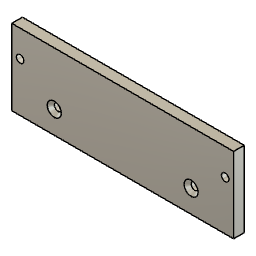
tip top audio zrail bracket (Autodesk Fusion 360 design; units mm, degrees)
Autodesk Fusion 360 part; units mm, degrees
note: some values were not read from the file. Set by a fixed rule: the direction of a hole.
sketch "Sketch2" plane through (0, 0, 0) normal (0, 0, 1) x (1, 0, 0)
  line L0 (-66.2534, 12.7) -> (66.2534, 12.7)
  line L1 (66.2534, 12.7) -> (66.2534, -12.7)
  line L2 (66.2534, -12.7) -> (-66.2534, -12.7)
  line L3 (-66.2534, -12.7) -> (-66.2534, 12.7)
  line L4 (-66.2534, 0) -> (66.2534, 0) construction
  line L5 (0, 12.7) -> (0, -12.7) construction
  line L6 (-66.2534, -12.7) -> (66.2534, -12.7)
  line L7 (66.2534, -12.7) -> (66.2534, -32.512)
  line L8 (66.2534, -32.512) -> (-66.2534, -32.512)
  line L9 (-66.2534, -32.512) -> (-66.2534, -12.7)
  point P0 (-61.2521, 0)
  point P1 (61.2521, 0)
  point P2 (-40.8534, -19.05)
  point P3 (-61.2521, -3.2004)
  point P4 (61.2521, -3.2004)
  point P5 (40.8534, -19.05)
  dimension "d2" = 25.4
  dimension "d3" = 122.5042
  dimension "d4" = 132.5067
  dimension "d18" = 3.2004
  dimension "d19" = 25.4
  dimension "d22" = 19.05
  dimension "d23" = 19.812
  constraint horizontal L0
  constraint vertical L1
  constraint horizontal L2
  constraint vertical L3
  constraint horizontal P0 P1
  constraint midpoint L3 L4.start
  constraint midpoint L1 L4.end
  constraint coincident P1 L4
  constraint midpoint L0 L5.start
  constraint midpoint L2 L5.end
  constraint symmetric P0 P1 L5
  constraint midpoint L4 origin
  constraint horizontal P3 P4
  constraint vertical P1 P4
  constraint vertical P0 P3
  constraint horizontal L6
  constraint vertical L7
  constraint horizontal L8
  constraint vertical L9
  constraint coincident L2.end L3.start
  constraint collinear L1 L7
  constraint symmetric L5 P2 P5
  measures "d2" distance of L0.start L2.end
  measures "d3" distance of P0 P1
  measures "d4" distance of L0.start L0.end
  measures "d18" distance of P0 P3
  measures "d19" distance of L3 P2
  measures "d22" distance of L4 P2
  measures "d23" distance of L6 L8
extrude "Extrude1" add sketch "Sketch2" along normal blind 6.35
hole "Hole1" at (-61.2521, -3.2004, 0) at (61.2521, -3.2004, 0) direction (0, 0, 1) diameter 4.4958 end through all
hole "Hole2" at (-40.8534, -19.05, 0) at (40.8534, -19.05, 0) direction (0, 0, 1) diameter 4.4958 depth 7.62 tip angle 118 countersink diameter 8.4328 countersink angle 82
move_body "Move1" bodies 1 to x (-1, 0, 0) y (0, 1, 0) z (0, 0, -1) at (0, 0, 0)
equation "d3 = tiptop_spacing"
equation "d4 = 5.125 in + ( ( 0.0459 * 2 ) * 1 in )"
equation "synthrotek_spacing = 4.741 in"
equation "tiptop_spacing = 4.823 in"
